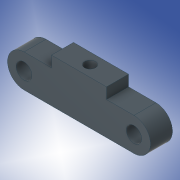
# Autodesk Inventor part: GA003
Saved by Autodesk Inventor 2017 (Build 210142000, 142)
## iProperties
Created: 2017-06-20
Part Number: GA003
Material: ABS Plastic
Document SubType Name: Modeling
Designer: zallen
Density: 1.06 g/cm^3
Appearance: CR Dark Blue
Author: zallen
Autodesk Inventor part; units mm, degrees
ref_plane "YZ Plane" through (0, 0, 0) normal (1, 0, 0) x (0, 1, 0)
ref_plane "XZ Plane" through (0, 0, 0) normal (0, 1, 0) x (-1, 0, 0)
ref_plane "XY Plane" through (0, 0, 0) normal (0, 0, 1) x (1, 0, 0)
sketch "Sketch1" plane through (0, 0, 0) normal (0, 0, 1) x (1, 0, 0)
  circle A0 centre (0, 0) radius 3.6
  circle A1 centre (0, 0) radius 7.5 construction
  arc A2 (0, 7.5) -> (0, -7.5) centre (0, 0) ccw
  line L0 (0, 7.5) -> (50, 7.5)
  line L1 (0, -7.5) -> (50, -7.5)
  circle A3 centre (50, 0) radius 7.5 construction
  arc A4 (50, -7.5) -> (50, 7.5) centre (50, 0) ccw
  circle A5 centre (50, 0) radius 3.5
  point P0 (42.6287, 1.3837)
  point P1 (42.5553, -0.9092)
  dimension "d0" = 7.2
  dimension "d1" = 15
  dimension "d2" = 50
  dimension "d3" = 15
  dimension "d4" = 7
  constraints: 10 point on circle, 6 centre point, 6 tangent, 4 end point, 3 coincident, 3 vertical alignment, 2 horizontal, 1 concentric
  measures "d0" diameter of A0
  measures "d1" diameter of A1
  measures "d2" distance of L0.start L0.end
  measures "d3" diameter of A3
  measures "d4" diameter of A5
extrude "Extrusion1" add sketch "Sketch1" along normal blind 10
sketch "Sketch4" plane through (0, 0, 10) normal (0, 0, 1) x (1, 0, 0)
  line L0 (50, 7.5) -> (0, 7.5) projected
  line L1 (12.5, 7.5) -> (37.5, 7.5)
  line L2 (37.5, 7.5) -> (37.5, 12.5)
  line L3 (37.5, 12.5) -> (12.5, 12.5)
  line L4 (12.5, 12.5) -> (12.5, 7.5)
  point P0 (0, 0)
  point P1 (25, 7.5)
  dimension "d10" = 25
  dimension "d11" = 5
  constraints: 8 end point, 2 midpoint, 2 parallel, 1 horizontal, 1 perpendicular, 1 point on line
  measures "d10" distance of L3.end L2.end
  measures "d11" distance of L3.end L1.start
extrude "Extrusion3" add sketch "Sketch4" against normal blind 10
sketch "Sketch5" plane through (12.5, 12.5, 10) normal (0, 1, 0) x (1, 0, 0)
  line L0 (25, 0) -> (0, 0) projected
  line L1 (25, 0) -> (25, 10) projected
  line L2 (0, 10) -> (25, 10) projected
  line L3 (0, 0) -> (0, 10) projected
  circle A0 centre (12.5, 5) radius 2.5
  line L4 (0, 0) -> (0, 10) projected
  point P0 (-12.5, 10)
  point P1 (12.5, 10)
  point P2 (0, 5)
  dimension "d14" = 5
  constraints: 2 midpoint, 1 centre point, 1 horizontal alignment, 1 vertical alignment
  measures "d14" diameter of A0
extrude "Extrusion4" cut sketch "Sketch5" against normal blind 10 contours A0
body "Solid1"
